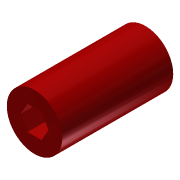
# Autodesk Inventor part: Part155
Saved by Autodesk Inventor 2014 SP2 (Build 180246200, 246)
## iProperties
Created: 2014-12-15
Part Number: Part155
Material: ABS Plastic
Document SubType Name: Modeling
Designer: Admin
Density: 1.06 g/cm^3
Appearance: Smooth - Red
Author: Admin
Autodesk Inventor part; units mm, degrees
ref_plane "YZ Plane" through (0, 0, 0) normal (1, 0, 0) x (0, 1, 0)
ref_plane "XZ Plane" through (0, 0, 0) normal (0, 1, 0) x (-1, 0, 0)
ref_plane "XY Plane" through (0, 0, 0) normal (0, 0, 1) x (1, 0, 0)
sketch "Sketch1" plane through (0, 0, 0) normal (0, 0, 1) x (1, 0, 0)
  arc A0 (-1.9939, 4.5894) -> (1.9939, 4.5894) centre (0, 0) ccw
  circle A1 centre (0, 0) radius 12.7
  line L0 (-1.9939, 4.5894) -> (-1.9939, 7.0024)
  line L1 (-1.9939, 7.0024) -> (1.9939, 7.0024)
  line L2 (1.9939, 7.0024) -> (1.9939, 4.5894)
  point P0 (0, 5.0038)
  dimension "d0" = 10.0076
  dimension "d1" = 25.4
  dimension "d5" = 2.413
  constraints: 6 end point, 3 point on circle, 2 centre point, 2 coincident, 1 parallel, 1 perpendicular
  measures "d0" diameter of A0
  measures "d1" diameter of A1
  measures "d5" distance of L0.start L0.end
extrude "Extrusion1" add sketch "Sketch1" along normal blind 25.4
sketch "Sketch2" plane through (0, 0, 25.4) normal (0, 0, 1) x (1, 0, 0)
  line L0 (-1.9939, 4.5894) -> (-1.9939, 7.0024) projected
  line L1 (-1.9939, 7.0024) -> (1.9939, 7.0024) projected
  line L2 (1.9939, 7.0024) -> (1.9939, 4.5894) projected
  arc A0 (-1.9939, 4.5894) -> (1.9939, 4.5894) centre (0, 0) ccw projected
  circle A1 centre (0, 0) radius 12.7 projected
  circle A2 centre (0, 0) radius 12.7
  line L3 (6.4158, 0) -> (3.2079, -5.5563)
  line L4 (3.2079, -5.5563) -> (-3.2079, -5.5563)
  line L5 (-3.2079, -5.5563) -> (-6.4158, 0)
  line L6 (-6.4158, 0) -> (-3.2079, 5.5562)
  line L7 (-3.2079, 5.5562) -> (3.2079, 5.5563)
  line L8 (3.2079, 5.5563) -> (6.4158, 0)
  line L9 (-1.9939, 7.0024) -> (1.9939, 7.0024)
  line L10 (1.9939, 7.0024) -> (1.9939, 5.5563)
  line L11 (1.9939, 5.5563) -> (-1.9939, 5.5563)
  line L12 (-1.9939, 5.5563) -> (-1.9939, 7.0024)
  dimension "d8" = 11.1125
  constraints: 20 end point, 2 coincident, 2 parallel, 2 point on line, 1 centre point, 1 concentric, 1 horizontal, 1 perpendicular, 13 other
  measures "d8" distance between parallel lines of L4 L7
extrude "Extrusion2" add sketch "Sketch2" along normal blind 25.4 contours L0 L1 L2 L7 | A1
body "Solid1"
